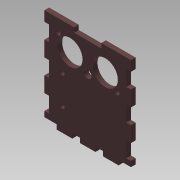
# Autodesk Inventor part: srfdiagkanan
Saved by Autodesk Inventor 2015 SP1 (Build 190203100, 203)
## iProperties
Created: 2015-02-13
Part Number: srfdiagkanan
Material: Generic
Document SubType Name: Modeling
Designer: Rafi Kurnia Putra
Density: 1 g/cm^3
Appearance: Default(2)
Author: Rafi Kurnia Putra
Autodesk Inventor part; units mm, degrees
ref_plane "YZ Plane" through (0, 0, 0) normal (1, 0, 0) x (0, 1, 0)
ref_plane "XZ Plane" through (0, 0, 0) normal (0, 1, 0) x (-1, 0, 0)
ref_plane "XY Plane" through (0, 0, 0) normal (0, 0, 1) x (1, 0, 0)
sketch "Sketch1" plane through (0, 0, 0) normal (0, 0, 1) x (1, 0, 0)
  line L0 (8.75, -28.5) -> (8.75, -31.5)
  line L1 (25.0209, -31.5) -> (8.75, -31.5)
  line L2 (-8.75, -28.5) -> (8.75, -28.5)
  circle A0 centre (11.43, -16.1838) radius 8.115
  circle A1 centre (19.05, -8.9448) radius 1.5875
  circle A2 centre (-19.05, -23.4228) radius 1.5875
  circle A3 centre (0, -9.5798) radius 2.5
  circle A4 centre (-11.43, -16.1838) radius 8.115
  line L3 (0, 8) -> (0, 18) construction
  line L4 (0, 18) -> (8.75, 18) construction
  line L5 (5, 31.5) -> (-5, 31.5)
  line L6 (-5, 28.5) -> (5, 31.5) construction
  line L7 (5, 28.5) -> (-5, 31.5) construction
  line L8 (-5, 28.5) -> (5, 28.5) construction
  line L9 (20, 31.5) -> (10, 31.5)
  line L10 (-10, 31.5) -> (-20, 31.5)
  line L11 (5, 31.5) -> (-5, 31.5)
  line L12 (-10, 28.5) -> (-10, 31.5)
  line L13 (-20, 28.5) -> (-20, 31.5)
  line L14 (10, 28.5) -> (10, 31.5)
  line L15 (20, 31.5) -> (20, 28.5)
  line L16 (-10, 28.5) -> (-5, 28.5)
  line L17 (5, 28.5) -> (10, 28.5)
  line L18 (-28.0209, -5) -> (-28.0209, -15)
  line L19 (-28.0209, -15) -> (-25.0209, -15)
  line L20 (-25.0209, -25) -> (-28.0209, -25)
  line L21 (-28.0209, -25) -> (-28.0209, -31.5)
  line L22 (-28.0209, -5) -> (-25.0209, -5)
  line L23 (-28.0209, 5) -> (-25.0209, 5)
  line L24 (-28.0209, 5) -> (-28.0209, 15)
  line L25 (-28.0209, 15) -> (-25.0209, 15)
  line L26 (-25.0209, 25) -> (-28.0209, 25)
  line L27 (-28.0209, 25) -> (-28.0209, 28.5)
  line L28 (-28.0209, 28.5) -> (-20, 28.5)
  line L29 (-25.0209, 15) -> (-25.0209, 25)
  line L30 (-25.0209, -25) -> (-25.0209, -15)
  line L31 (-25.0209, -5) -> (-25.0209, 5)
  line L32 (28.0209, -5) -> (28.0209, -15)
  line L33 (28.0209, -15) -> (25.0209, -15)
  line L34 (25.0209, -25) -> (28.0209, -25)
  line L35 (28.0209, -25) -> (28.0209, -31.5)
  line L36 (28.0209, -31.5) -> (25.0209, -31.5)
  line L37 (28.0209, -5) -> (25.0209, -5)
  line L38 (28.0209, 5) -> (25.0209, 5)
  line L39 (28.0209, 5) -> (28.0209, 15)
  line L40 (28.0209, 15) -> (25.0209, 15)
  line L41 (25.0209, 25) -> (28.0209, 25)
  line L42 (28.0209, 25) -> (28.0209, 28.5)
  line L43 (28.0209, 28.5) -> (20, 28.5)
  line L44 (25.0209, 15) -> (25.0209, 25)
  line L45 (25.0209, -25) -> (25.0209, -15)
  line L46 (25.0209, -5) -> (25.0209, 5)
  line L47 (-8.75, -31.5) -> (-8.75, -28.5)
  line L48 (-28.0209, -31.5) -> (-8.75, -31.5)
  line L49 (-5, 28.5) -> (-5, 31.5)
  line L50 (5, 28.5) -> (5, 31.5)
  circle A5 centre (-16.4791, 16.5) radius 1.5
  circle A6 centre (-16.4791, -2.25) radius 1.5
  point P0 (0, 0)
  point P1 (0, 30)
  dimension "d2" = 3
  dimension "d5" = 15
  dimension "d8" = 15
  dimension "d12" = 5
  dimension "d13" = 10
  dimension "d16" = 3
  dimension "d17" = 3
  constraints: 102 end point, 17 perpendicular, 14 symmetric about line, 9 vertical, 8 point on line, 7 centre point, 6 horizontal, 3 equal length, 2 midpoint, 10 other
  measures "d2" distance of L5.start L7.start
  measures "d5" distance of L5.start L9.start
  measures "d8" distance of L5.start L10.start
  measures "d12" vertical distance of point (0, 0) L18.start
  measures "d13" distance of L18.start L18.end
  measures "d16" distance of L20.start L20.end
  measures "d17" distance of L23.start L23.end
extrude "Extrusion3" add sketch "Sketch1" along normal mid plane 3
body "Solid3"
